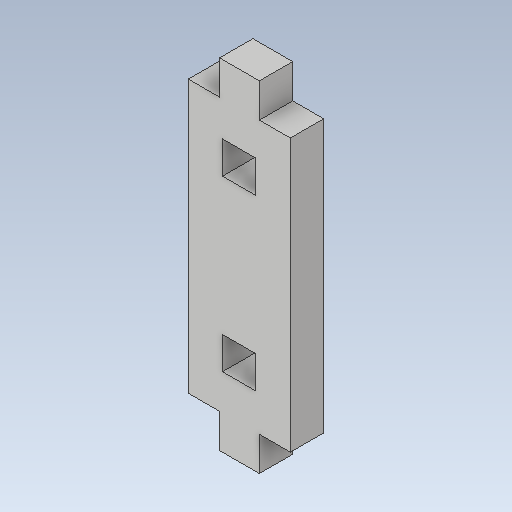
# Autodesk Inventor part: В. шарн. - соединитель
Saved by Autodesk Inventor 2020 (Build 240168000, 168)
## iProperties
Created: 2020-02-22
Part Number: В. шарн. - соединитель
Material: Типовые
Document SubType Name: Modeling
Designer: Leancher
Density: 1 g/cm^3
Appearance: По умолчанию
Author: Leancher
Autodesk Inventor part; units mm, degrees
ref_plane "YZ Plane" through (0, 0, 0) normal (1, 0, 0) x (0, 1, 0)
ref_plane "XZ Plane" through (0, 0, 0) normal (0, 1, 0) x (-1, 0, 0)
ref_plane "XY Plane" through (0, 0, 0) normal (0, 0, 1) x (1, 0, 0)
sketch "Эскиз1" plane through (0, 0, 0) normal (0, 0, 1) x (1, 0, 0)
  line L0 (2.2305, 14.4712) -> (2.2305, 9.7212)
  line L1 (2.2305, 9.7212) -> (-2.6195, 9.7212)
  line L2 (-2.6195, 9.7212) -> (-2.6195, 14.4712)
  line L3 (-2.6195, 14.4712) -> (2.2305, 14.4712)
  line L4 (7.3598, -20.4288) -> (7.3598, 19.5712)
  line L5 (7.3598, 19.5712) -> (2.8055, 19.5712)
  line L6 (2.8055, 19.5712) -> (2.8055, 24.5712)
  line L7 (2.8055, 24.5712) -> (-3.0445, 24.5712)
  line L8 (-3.0445, 24.5712) -> (-3.0445, 19.5712)
  line L9 (-3.0445, 19.5712) -> (-7.6402, 19.5712)
  line L10 (-7.6402, 19.5712) -> (-7.6402, -20.4288)
  line L11 (-7.6402, -20.4288) -> (-3.0445, -20.4288)
  line L12 (-3.0445, -20.4288) -> (-3.0445, -25.4288)
  line L13 (-3.0445, -25.4288) -> (2.8055, -25.4288)
  line L14 (2.8055, -25.4288) -> (2.8055, -20.4288)
  line L15 (2.8055, -20.4288) -> (7.3598, -20.4288)
  line L16 (2.2305, -10.4288) -> (2.2305, -15.1788)
  line L17 (2.2305, -15.1788) -> (-2.6195, -15.1788)
  line L18 (-2.6195, -15.1788) -> (-2.6195, -10.4288)
  line L19 (-2.6195, -10.4288) -> (2.2305, -10.4288)
  constraints: 40 end point
extrude "Выдавливание1" add sketch "Эскиз1" along normal blind 4.9
